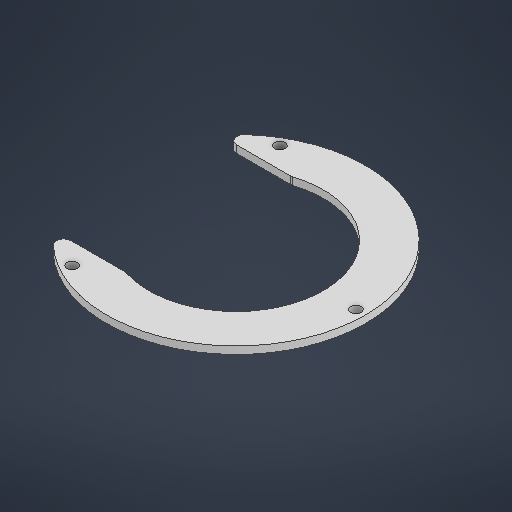
# Autodesk Inventor part: Cylinder Segment Holder
Saved by Autodesk Inventor 2026.1 (Build 301233000, 233)
## iProperties
Created: 2025-02-13
Part Number: Cylinder Segment Holder
Material: Generic
Document SubType Name: Modeling
Designer: mayhe
Density: 1 g/cm^3
Appearance: Default
Author: mayhe
Autodesk Inventor part; units mm, degrees
ref_plane "YZ Plane" through (0, 0, 0) normal (1, 0, 0) x (0, 1, 0)
ref_plane "XZ Plane" through (0, 0, 0) normal (0, 1, 0) x (-1, 0, 0)
ref_plane "XY Plane" through (0, 0, 0) normal (0, 0, 1) x (1, 0, 0)
sketch "Sketch1" plane through (0, 0, 0) normal (0, 1, 0) x (-1, 0, 0)
  circle A0 centre (0, 0) radius 59
  circle A1 centre (0, 0) radius 81
  circle A2 centre (0, 0) radius 87.5
  line L0 (90, -56) -> (15, -56)
  line L1 (10, -51) -> (10, 51)
  line L2 (15, 56) -> (90, 56)
  line L3 (90, 56) -> (90, -56)
  line L4 (90, -56) -> (10, 56) construction
  line L5 (10, -56) -> (90, 56) construction
  arc A3 (10, -51) -> (15, -56) centre (15, -51) ccw
  arc A4 (15, 56) -> (10, 51) centre (15, 51) ccw
  point P0 (50, 0)
  point P1 (90, 0)
  point P2 (10, 0)
  point P3 (60, -54.4151)
  point P4 (60, 54.4151)
  point P5 (80, 35.4436)
  point P6 (80, -35.4436)
  point P7 (67.2328, 56)
  point P8 (67.2328, -56)
  dimension "d0" = 118
  dimension "d1" = 162
  dimension "d2" = 175
  dimension "d7" = 112
  dimension "d9" = 80
  dimension "d10" = 10
  dimension "d11" = 5
  constraints: 12 end point, 5 centre point, 4 midpoint, 4 point on circle, 4 point on line, 4 tangent, 3 coincident, 2 parallel, 1 equal radius, 1 horizontal, 1 perpendicular
  measures "d0" diameter of A0
  measures "d1" diameter of A1
  measures "d2" diameter of A2
  measures "d7" distance of L4.end L5.start
  measures "d9" distance of L4.end L2.end
  measures "d10" distance of point (0, 0) point (10, 0)
  measures "d11" radius of A3
extrude "Extrusion1" add sketch "Sketch1" along normal blind 5 contours A0 L0 A1 L2 | A1 L0 A2 L2 picked at (42.125, 58.7621) picked at (-85.0936, 2.0693)
fillet "Fillet1" radius 5 4 edges at (-67.2328, 2.5, -56) (-67.2328, 2.5, 56) (-18.5742, 2.5, -56) (-18.5742, 2.5, 56)
sketch "Sketch2" plane through (0, 5, 0) normal (0, 1, 0) x (1, 0, 0)
  circle A0 centre (0, 0) radius 70.375
  line L0 (-36.4414, 79.1184) -> (-50.2978, 71.1184)
  line L1 (-50.2978, 71.1184) -> (-44.9056, 61.7788)
  arc A1 (-31.0492, 69.7788) -> (-44.9056, 61.7788) centre (0, 0) ccw
  line L2 (-31.0492, 69.7788) -> (-36.4414, 79.1184)
  circle A2 centre (-40.5, 70.1481) radius 3.5625
  circle A3 centre (-40.5, 70.1481) radius 3.5625
  line L3 (86.7392, -8) -> (86.7392, 8)
  line L4 (86.7392, 8) -> (75.9549, 8)
  arc A4 (75.9549, -8) -> (75.9549, 8) centre (0, 0) ccw
  line L5 (75.9549, -8) -> (86.7392, -8)
  arc A5 (80.9215, -3.5651) -> (80.9217, -3.5616) centre (0, 0) ccw
  arc A6 (81.0783, -3.5616) -> (80.9217, -3.5616) centre (81, 0) ccw
  line L6 (81.0783, -3.5616) -> (80.9215, -3.5651)
  line L7 (-50.2978, -71.1184) -> (-36.4414, -79.1184)
  line L8 (-36.4414, -79.1184) -> (-31.0492, -69.7788)
  arc A7 (-44.9056, -61.7788) -> (-31.0492, -69.7788) centre (0, 0) ccw
  line L9 (-44.9056, -61.7788) -> (-50.2978, -71.1184)
  circle A8 centre (-40.5, -70.1481) radius 3.5625
  point P0 (-65.1143, 450.6181)
  constraints: 20 end point, 10 point on circle, 9 centre point
extrude "Extrusion2" cut sketch "Sketch2" against normal blind 10 contours A2 | A5 A6 L6 | A8
body "Solid1"
